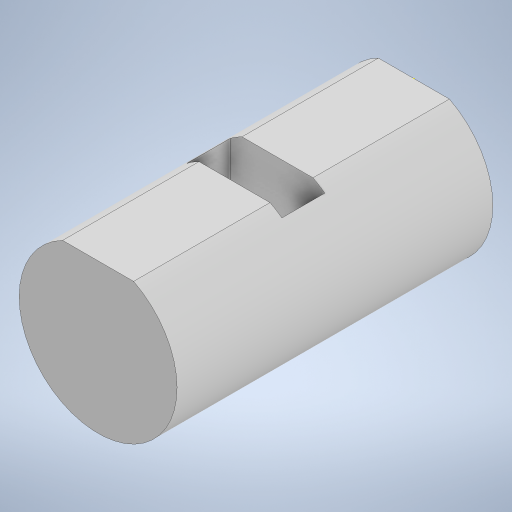
# Autodesk Inventor part: foot
Saved by Autodesk Inventor 2023 (Build 270158000, 158)
## iProperties
Created: 2022-12-19
Part Number: foot
Material: Generic
Document SubType Name: Modeling
Designer: LAB-505
Density: 1.01292 g/cm^3
Appearance: Default
Mass: 22 g
Surface Area: 56.0563 cm^2
Volume: 21.7194 cm^3
Author: LAB-505
Autodesk Inventor part; units mm, degrees
ref_plane "YZ Plane" through (0, 0, 0) normal (1, 0, 0) x (0, 1, 0)
ref_plane "XZ Plane" through (0, 0, 0) normal (0, 1, 0) x (-1, 0, 0)
ref_plane "XY Plane" through (0, 0, 0) normal (0, 0, 1) x (1, 0, 0)
sketch "Sketch12" plane through (0, 0, 0) normal (0, 0, 1) x (1, 0, 0)
  circle A0 centre (0, 0) radius 12.5
  dimension "d22" = 25
  constraints: 1 centre point, 1 coincident
  measures "d22" diameter of A0
extrude "Extrusion3" add sketch "Sketch12" along normal blind 50
sketch "Sketch15" plane through (0, 0, 50) normal (0, 0, 1) x (1, 0, 0)
  circle A0 centre (0, 0) radius 12.5 projected
  line L0 (-5.6199, 11.1654) -> (6.24, 11.1654)
  line L1 (6.24, 11.1654) -> (6.24, 16.8143)
  line L2 (6.24, 16.8143) -> (-5.6199, 16.8143)
  line L3 (-5.6199, 16.8143) -> (-5.6199, 11.1654)
  constraints: 8 end point, 2 parallel, 1 horizontal, 1 perpendicular, 2 other
extrude "Extrusion4" cut sketch "Sketch15" against normal blind 64.3 contours L3 L2 L1 L0 A0 | A0 L0 picked at (0.9627, 11.4975)
sketch "Sketch17" plane through (-5.6199, 11.1654, 50) normal (0, 1, 0) x (1, 0, 0)
  point P0 (5.6199, 50)
sketch "Sketch18" plane through (-5.6199, 11.1654, 50) normal (0, 1, 0) x (1, 0, 0)
  line L0 (-1.8801, 28.4) -> (13.1199, 28.4)
  line L1 (13.1199, 28.4) -> (13.1199, 21.6)
  line L2 (13.1199, 21.6) -> (-1.8801, 21.6)
  line L3 (-1.8801, 21.6) -> (-1.8801, 28.4)
  line L4 (-1.8801, 28.4) -> (13.1199, 21.6) construction
  line L5 (13.1199, 28.4) -> (-1.8801, 21.6) construction
  point P0 (5.6199, 50)
  point P1 (5.6199, 25)
  dimension "d30" = 15
  dimension "d31" = 6.8
  constraints: 12 end point, 2 midpoint, 2 parallel, 1 horizontal, 1 perpendicular
  measures "d30" distance of L1.end L2.end
  measures "d31" distance of L0.end L1.end
extrude "Extrusion6" cut sketch "Sketch18" against normal blind 28.2625
body "Solid7"
